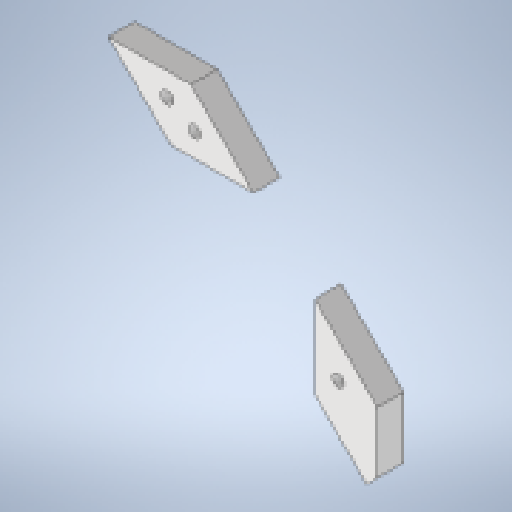
# Autodesk Inventor part: Dribbler_v1
Saved by Autodesk Inventor 2025.1 (Build 291241000, 241)
## iProperties
Created: 2026-05-04
Part Number: Dribbler_v1
Material: Generic
Document SubType Name: Modeling
Designer: User
Density: 1 g/cm^3
Appearance: Default
Author: User
## iProperties of the stored document Dribbler_v1_3DPrint.ipt
Created: 2026-05-05
Part Number: Dribbler_v1_3DPrint
Material: Generic
Document SubType Name: Modeling
Designer: User
Density: 1 g/cm^3
Appearance: Default
Author: User
Autodesk Inventor part; units mm, degrees
ref_plane "YZ Plane" through (0, 0, 0) normal (1, 0, 0) x (0, 1, 0)
ref_plane "XZ Plane" through (0, 0, 0) normal (0, 1, 0) x (-1, 0, 0)
ref_plane "XY Plane" through (0, 0, 0) normal (0, 0, 1) x (1, 0, 0)
sketch "Sketch1" plane through (0, 0, 0) normal (0, 0, 1) x (1, 0, 0)
  circle A0 centre (-1.926, 3.4009) radius 1.5 projected
  circle A1 centre (1.926, -3.4009) radius 1.5 projected
  line L0 (5.5, -12.5711) -> (5.5, 1.5711) projected
  line L1 (5.5, 1.5711) -> (-5.5, 12.5711) projected
  line L2 (-5.5, 12.5711) -> (-5.5, -1.5711) projected
  line L3 (-5.5, -1.5711) -> (5.5, -12.5711) projected
  circle A2 centre (-44.1118, 42.6369) radius 1.5 projected
  circle A3 centre (-37.31, 38.7849) radius 1.5 projected
  line L4 (-53.282, 46.2109) -> (-42.282, 35.2109) projected
  line L5 (-42.282, 35.2109) -> (-28.1398, 35.2109) projected
  line L6 (-28.1398, 35.2109) -> (-39.1398, 46.2109) projected
  line L7 (-39.1398, 46.2109) -> (-53.282, 46.2109) projected
  line L8 (-5.7, 13.0539) -> (5.7, 1.6539)
  line L9 (5.7, 1.6539) -> (5.7, -13.0539)
  line L10 (5.7, -13.0539) -> (-5.7, -1.6539)
  line L11 (-5.7, -1.6539) -> (-5.7, 13.0539)
  line L12 (-27.657, 35.0109) -> (-42.3648, 35.0109)
  line L13 (-42.3648, 35.0109) -> (-53.7648, 46.4109)
  line L14 (-53.7648, 46.4109) -> (-39.057, 46.4109)
  line L15 (-39.057, 46.4109) -> (-27.657, 35.0109)
  line L16 (-7.7, -2.4823) -> (7.7, -17.8823)
  line L17 (7.7, -17.8823) -> (7.7, 2.4823)
  line L18 (7.7, 2.4823) -> (-7.7, 17.8823)
  line L19 (-7.7, 17.8823) -> (-7.7, -2.4823)
  line L20 (-43.1932, 33.0109) -> (-22.8285, 33.0109)
  line L21 (-22.8285, 33.0109) -> (-38.2285, 48.4109)
  line L22 (-38.2285, 48.4109) -> (-58.5932, 48.4109)
  line L23 (-58.5932, 48.4109) -> (-43.1932, 33.0109)
  point P0 (0, 0)
  dimension "d0" = 0.2
  dimension "d1" = 0.2
  dimension "d2" = 2
  dimension "d3" = 2
  constraints: 32 end point, 12 other
  measures "d0" distance between parallel lines of L1 L8
  measures "d1" distance between parallel lines of L5 L12
  measures "d2" distance between parallel lines of L10 L16
  measures "d3" distance between parallel lines of L12 L20
ref_plane "Work Plane1" through (-5.5, -57.7526, -4) normal (0, 0, 1) x (1, 0, 0)
extrude "Extrusion1" add sketch "Sketch1" against normal up to surface (4 mm away) contours L19 L18 L17 L16 | L23 L22 L21 L20
sketch "Sketch2" plane through (0, 0, 0) normal (0, 0, 1) x (1, 0, 0)
  line L0 (-7.7, 17.8823) -> (-7.7, -2.4823) projected
  line L1 (7.7, 2.4823) -> (-7.7, 17.8823) projected
  line L2 (-7.7, -2.4823) -> (7.7, -17.8823) projected
  line L3 (7.7, -17.8823) -> (7.7, 2.4823) projected
  line L4 (-43.1932, 33.0109) -> (-22.8285, 33.0109) projected
  line L5 (-58.5932, 48.4109) -> (-43.1932, 33.0109) projected
  line L6 (-22.8285, 33.0109) -> (-38.2285, 48.4109) projected
  line L7 (-38.2285, 48.4109) -> (-58.5932, 48.4109) projected
  point P0 (0, 0)
extrude "Extrusion2" add sketch "Sketch2" along normal blind 2.5
sketch "Sketch3" plane through (0, 0, 2.5) normal (0, 0, 1) x (1, 0, 0)
  circle A0 centre (-44.1118, 42.6369) radius 1.5 projected
  circle A1 centre (-37.31, 38.7849) radius 1.5 projected
  circle A2 centre (-1.926, 3.4009) radius 1.5 projected
  point P0 (0, 0)
extrude "Extrusion3" cut sketch "Sketch3" against normal blind 2.5
sketch "Sketch34" plane through (0, 0, 2.5) normal (0, 0, 1) x (1, 0, 0)
  line L0 (12.8478, -6.0634) -> (8.0273, -10.8596)
  line L1 (7.7, -17.8823) -> (7.7, 2.4823) projected
  line L2 (-7.7, -2.4823) -> (7.7, -17.8823) projected
  line L3 (13.5531, -6.7723) -> (8.7326, -11.5685)
  line L4 (7.7, -12.5958) -> (5.0567, -15.2391)
  point P0 (0, 0)
  dimension "d105" = 1
  constraints: 6 end point, 2 point on line, 1 parallel, 1 perpendicular, 3 other
  measures "d105" distance between parallel lines of L0 L3
extrude "Extrusion31" cut sketch "Sketch34" against normal blind 10
sketch "Sketch36" plane through (0, 0, 2.5) normal (0, 0, 1) x (1, 0, 0)
  circle A0 centre (1.926, -3.4009) radius 1.5
  point P0 (0, 0)
  constraints: 1 centre point, 2 other
extrude "Extrusion32" cut sketch "Sketch36" against normal blind 10
sketch "Sketch37" plane through (-7.7, 17.8823, 2.5) normal (0.7071068, 0.7071068, 0) x (0, 0, -1)
  line L0 (1.1916, -14.1408) -> (1.1916, -32.4408)
  line L1 (1.6916, -14.1408) -> (1.6916, -32.4408)
  line L2 (6.5, -21.7789) -> (0, -21.7789) projected
  line L3 (6.5, 0) -> (6.5, -21.7789) projected
  line L4 (1.3722, -14.1408) -> (4.885, -14.1408)
  line L5 (1.6916, -21.7789) -> (6.5, -21.7789)
  line L6 (6.5, -21.7789) -> (6.5, -14.1408)
  line L7 (6.5, -14.1408) -> (1.6916, -14.1408)
  line L8 (1.6916, -14.1408) -> (1.6916, -21.7789)
  point P0 (2.5, -18.0894)
  point P1 (4.885, -14.1408)
  dimension "d110" = 0.5
  constraints: 14 end point, 3 parallel, 3 point on line, 2 horizontal, 1 perpendicular, 1 vertical, 4 other
  measures "d110" distance between parallel lines of L0 L1
extrude "Extrusion33" add sketch "Sketch37" along normal blind 19
sketch "Sketch38" plane through (7.7, 2.4823, -4) normal (0.7071068, -0.7071068, 0) x (0.7071068, 0.7071068, 0)
  line L0 (16.4612, 13.1005) -> (7.0738, 5.3084)
  line L1 (16.7806, 12.7158) -> (7.3931, 4.9237)
  line L2 (0, 4.8084) -> (19, 4.8084) projected
  line L3 (7.3931, 4.9237) -> (7.2543, 4.8084)
  line L4 (0, 4.8084) -> (19, 4.8084) projected
  line L5 (19, 4.8084) -> (19, 0) projected
  line L6 (16.4612, 13.1005) -> (19.5269, 9.4071)
  line L7 (19, 4.8084) -> (19, 10.0419)
  line L8 (19, 4.8084) -> (24.2335, 4.8084) construction
  arc A0 (14.4327, 6.933) -> (13.5093, 6.1666) centre (13.46, 7.1654) ccw
  circle A1 centre (13.46, 7.1654) radius 1
  point P0 (-7.2, 4)
  point P1 (14.4327, 6.933)
  point P2 (13.5093, 6.1666)
  dimension "d113" = 0.5
  dimension "d114" = 90
  constraints: 12 end point, 2 centre point, 2 point on circle, 2 point on line, 1 coincident, 1 concentric, 1 horizontal, 1 parallel, 1 perpendicular, 9 other
  measures "d113" distance between parallel lines of L0 L1
  measures "d114" angle of L8 L7
extrude "Extrusion34" add sketch "Sketch38" against normal up to surface (7.6381 mm away)
sketch "Sketch39" plane through (7.7, 2.4823, -4) normal (0.7071068, -0.7071068, 0) x (0.7071068, 0.7071068, 0)
  line L0 (7.0738, 5.3084) -> (-7.4246, 22.7752)
  line L1 (6.6891, 4.9891) -> (-7.8093, 22.4559)
  line L2 (0, 4.8084) -> (7.2543, 4.8084) projected
  line L3 (0, 4.8084) -> (0, 6.5) projected
  line L4 (-10.6619, 6.5) -> (0, 6.5) projected
  line L5 (6.6891, 4.9891) -> (6.839, 4.8084)
  line L6 (-4.6571, 4) -> (-4.6571, -2.5)
  line L7 (-4.6571, 6.5) -> (-4.6571, 4) projected
  line L8 (-4.6571, 4.8084) -> (-4.6571, 18.6583)
  point P0 (-7.2, 4)
  point P1 (-4.6571, 6.5)
  dimension "d117" = 0.5
  constraints: 10 end point, 3 point on line, 1 collinear, 1 parallel, 1 vertical, 5 other
  measures "d117" distance between parallel lines of L0 L1
extrude "Extrusion35" add sketch "Sketch39" against normal up to surface (7.6381 mm away)
sketch "Sketch40" plane through (0, 0, 2.5) normal (0, 0, 1) x (1, 0, 0)
  circle A0 centre (-1.926, 3.4009) radius 1.5 projected
  point P0 (0, 0)
  point P1 (-0.8654, 4.4616)
  constraints: 1 other
ref_plane "Work Plane4" through (-5.5, -12.5711, 0) normal (0, 0, 1) x (1, 0, 0)
extrude "Extrusion36" add sketch "Sketch40" against normal up to surface (2.5 mm away)
sketch "Sketch41" plane through (2.299, 7.8833, 2.5) normal (-0.7071068, 0.7071068, 0) x (0.7071068, 0.7071068, 0)
  line L0 (-7.4246, -16.2752) -> (1.9629, -24.0673)
  line L1 (-7.7439, -16.6599) -> (1.6435, -24.452)
  line L2 (6.839, 1.6916) -> (-4.6571, -12.1583) projected
  line L3 (-4.6571, -12.1583) -> (-4.6571, 0) projected
  line L4 (-4.6571, -12.1583) -> (-8.1286, -16.3406)
  line L5 (-8.1286, -16.3406) -> (-7.7439, -16.6599)
  arc A0 (-4.4727, -23.2091) -> (-5.396, -22.4427) centre (-4.4234, -22.2103) ccw
  circle A1 centre (-4.4234, -22.2103) radius 1
  line L6 (-5.3349, -24.2479) -> (-1.1029, -27.7607)
  line L7 (-10.4903, -19.9686) -> (-6.2583, -23.4814)
  line L8 (-5.9736, -25.0173) -> (-1.7416, -28.5301)
  line L9 (-11.129, -20.7381) -> (-6.897, -24.2509)
  line L10 (-1.1029, -27.7607) -> (1.9629, -24.0673)
  line L11 (1.6435, -24.452) -> (-1.7416, -28.5301)
  line L12 (-1.7416, -28.5301) -> (-11.5137, -20.4187)
  line L13 (0, 0) -> (-14.4, 0) projected
  line L14 (-11.5137, -20.4187) -> (-11.5137, 0)
  point P0 (-7.2, 2.5)
  point P1 (-4.4727, -23.2091)
  point P2 (-5.396, -22.4427)
  point P3 (-11.129, -20.7381)
  point P4 (-6.897, -24.2509)
  point P5 (-5.9736, -25.0173)
  point P6 (-1.1029, -27.7607)
  dimension "d122" = 0.5
  dimension "d123" = 1
  dimension "d124" = 1
  constraints: 24 end point, 4 perpendicular, 3 parallel, 2 centre point, 2 point on circle, 1 coincident, 1 concentric, 1 point on line, 14 other
  measures "d122" distance between parallel lines of L0 L1
  measures "d123" distance between parallel lines of L6 L8
  measures "d124" distance between parallel lines of L7 L9
extrude "Extrusion37" add sketch "Sketch41" against normal up to surface (7.6381 mm away)
sketch "Sketch42" plane through (0, 0, 2.5) normal (0, 0, 1) x (1, 0, 0)
  arc A0 (0.8121, -4.4055) -> (2.9306, -2.287) centre (1.926, -3.4009) ccw projected
  circle A1 centre (1.926, -3.4009) radius 3
  line L0 (0.8121, -4.4055) -> (-0.4414, -5.6591) projected
  line L1 (-0.4414, -5.6591) -> (-5.8424, -0.2581) projected
  line L2 (1.926, -3.4009) -> (4.0473, -5.5222)
  line L3 (1.926, -3.4009) -> (4.926, -3.4009) construction
  line L4 (4.0473, -5.5222) -> (-0.1953, -1.2796)
  line L5 (-0.1953, -1.2796) -> (-2.5081, -3.5924)
  point P0 (0, 0)
  point P1 (2.9867, -4.4616)
  dimension "d127" = 6
  dimension "d128" = 45
  constraints: 8 end point, 3 point on line, 2 point on circle, 1 centre point, 1 coincident, 1 equal length, 1 horizontal, 1 tangent
  measures "d127" diameter of A1
  measures "d128" angle of L2 L3
extrude "Extrusion38" cut sketch "Sketch42" along normal through all contours L0 A1 L4 L2 A0 | L2 L4 A1 | L0 L1 L5 A1
sketch "Sketch43" plane through (-5.8424, -0.2581, 22.9187) normal (-0.4516248, -0.4516248, 0.7694609) x (0.544091, 0.544091, 0.638694)
  line L0 (8.1483, -7.6381) -> (12.7, -7.6381) projected
  line L1 (0, -4.7154) -> (4.2508, -4.7154) projected
  line L2 (12.7, -7.6381) -> (0, -7.6381)
  line L3 (0, -7.6381) -> (0, -4.7154)
  line L4 (0, -4.7154) -> (12.7, -4.7154)
  line L5 (12.7, -4.7154) -> (12.7, -7.6381)
  point P0 (-11.3188, -3.9487)
  point P1 (8.1483, -7.6381)
  point P2 (4.2508, -4.7154)
  constraints: 8 end point, 2 parallel, 1 horizontal, 1 perpendicular
extrude "Extrusion39" cut sketch "Sketch43" against normal blind 10
sketch "Sketch44" plane through (2.299, 7.8833, 2.5) normal (-0.7071068, 0.7071068, 0) x (0.7071068, 0.7071068, 0)
  line L0 (-11.5137, 0) -> (-11.5137, -20.4187) projected
  line L1 (0, 0) -> (-14.4, 0) projected
  line L2 (-11.5137, -20.4187) -> (-1.7416, -28.5301) projected
  line L3 (-14.4, 6.5) -> (-14.4, 0) projected
  line L4 (-14.4, 0) -> (-14.4, -18.023)
  line L5 (-14.4, -18.023) -> (-11.5137, -20.4187)
  point P0 (-7.2, 2.5)
  constraints: 4 end point, 1 vertical
extrude "Extrusion40" add sketch "Sketch44" against normal up to surface (4.7154 mm away)
sketch "Sketch45" plane through (0, 0, 2.5) normal (0, 0, 1) x (1, 0, 0)
  line L0 (-7.8833, -2.299) -> (1.0675, 6.6518) projected
  line L1 (-7.7, 17.8823) -> (-7.7, -2.1157) projected
  line L2 (-1.5165, 4.0677) -> (-3.4257, 5.9769)
  line L3 (-1.5165, 4.0677) -> (-3.6379, 1.9464)
  line L4 (-3.6379, 1.9464) -> (-9.8213, 8.1299)
  line L5 (-9.8213, 8.1299) -> (-7.7, 10.2512)
  line L6 (-7.7, 10.2512) -> (-1.5165, 4.0677)
  point P0 (0, 0)
  point P1 (-7.7, 6.0086)
  dimension "d135" = 3
  constraints: 10 end point, 2 parallel, 1 perpendicular, 1 point on line, 3 other
  measures "d135" distance of L2.start L3.end
extrude "Extrusion41" add sketch "Sketch45" along normal up to surface contours L4 L1 L6 L2 L0 surface through (4.4069, -0.8107, 14.6583) normal (0.544091, 0.544091, 0.638694)
sketch "Sketch46" plane through (-7.7, -2.4823, -4) normal (0, 0, -1) x (-1, 0, 0)
  line L0 (0, 0) -> (0, 20.3647) projected
  line L1 (-2, 15.5362) -> (-2, 0.8284) projected
  line L2 (-12.7567, -12.7567) -> (0, 0) projected
  line L3 (0, 20.3647) -> (-9.999, 10.3657) projected
  line L4 (-2.0031, 18.3616) -> (-2, -2)
  line L5 (35.4932, 35.4932) -> (50.8932, 50.8932) projected
  line L6 (15.1285, 35.4932) -> (35.4932, 35.4932) projected
  line L7 (34.6648, 37.4932) -> (19.957, 37.4932) projected
  line L8 (30.5285, 50.8932) -> (15.1285, 35.4932) projected
  line L9 (37.4692, 37.4692) -> (17.1285, 37.4932)
  point P0 (-7.7, 2.4823)
  constraints: 6 point on line, 4 end point
extrude "Extrusion42" add sketch "Sketch46" along normal blind 5
sketch "Sketch47" plane through (0, 0, 2.5) normal (0, 0, 1) x (1, 0, 0)
  line L0 (5.5, -57.7526) -> (5.5, -12.5711)
  line L1 (-7.7, 6.0086) -> (-7.7, -2.1157) projected
  line L2 (-4.549, -5.6333) -> (5.0567, -15.2391) projected
  line L3 (5.0567, -15.2391) -> (5.0567, -34.2391)
  line L4 (5.0567, -34.2391) -> (-7.7, -34.2391)
  line L5 (-7.7, -34.2391) -> (-7.7, -2.1157)
  line L6 (5.0567, -15.2391) -> (7.7, -12.5958) projected
  line L7 (-7.8833, -2.299) -> (-4.549, -5.6333) projected
  point P0 (0, 0)
  point P1 (-7.7, -2.4823)
  dimension "d140" = 19
  dimension "d141" = 90
  constraints: 8 end point, 1 collinear, 1 parallel, 1 vertical, 2 other
  measures "d140" distance of L2.end L3.end
  measures "d141" angle of L3 L4
extrude "Extrusion43" add sketch "Sketch47" against normal up to surface (6.5 mm away)
sketch "Sketch48" plane through (0, 0, 2.5) normal (0, 0, 1) x (1, 0, 0)
  line L0 (-53.282, 46.2109) -> (-98.4635, 46.2109)
  line L1 (-38.2285, 48.4109) -> (-58.5932, 48.4109) projected
  line L2 (-58.5932, 48.4109) -> (-43.1932, 33.0109) projected
  line L3 (-56.3932, 46.2109) -> (-54.1932, 48.4109)
  line L4 (-56.3932, 46.2109) -> (-53.282, 46.2109) construction
  line L5 (-56.3932, 46.2109) -> (-55.6861, 45.5038)
  line L6 (-55.6861, 45.5038) -> (-52.779, 48.4109)
  point P0 (0, 0)
  dimension "d144" = 45
  dimension "d145" = 1
  constraints: 10 end point, 5 point on line, 2 horizontal, 1 equal length, 1 perpendicular, 2 other
  measures "d144" angle of L4 L3
  measures "d145" distance of L3.start L5.end
extrude "Extrusion44" cut sketch "Sketch48" against normal blind 10
sketch "Sketch50" plane through (0, 0, 2.5) normal (0, 0, 1) x (1, 0, 0)
  line L0 (-43.1932, 33.0109) -> (-22.8285, 33.0109) projected
  line L1 (-55.6861, 45.5038) -> (-43.1932, 33.0109) projected
  line L2 (-53.282, 46.2109) -> (-98.4635, 46.2109)
  line L3 (-7.7, -2.4823) -> (-7.7, -34.2391) projected
  line L4 (-55.6861, 45.5038) -> (-88.933, 45.5038)
  line L5 (-7.7, -34.2391) -> (-87.4429, 45.5038)
  line L6 (-7.7, -34.2391) -> (105.0734, -34.2391) construction
  line L7 (-22.8285, 33.0109) -> (-74.95, 33.0109)
  point P0 (0, 0)
  dimension "d148" = 135
  constraints: 10 end point, 3 horizontal, 2 point on line, 1 equal length, 1 parallel, 2 other
  measures "d148" angle of L6 L5
extrude "Extrusion45" add sketch "Sketch50" against normal up to surface (6.5 mm away)
sketch "Sketch51" plane through (0, 0, 2.5) normal (0, 0, 1) x (1, 0, 0)
  line L0 (-7.7, -34.2391) -> (5.0567, -34.2391) projected
  line L1 (-87.4429, 45.5038) -> (-74.95, 33.0109) projected
  line L2 (-7.7, -34.2391) -> (5.0567, -46.9958)
  line L3 (-7.7, -34.2391) -> (10.3408, -34.2391) construction
  line L4 (5.0567, -46.9958) -> (5.0567, -34.2391)
  point P0 (0, 0)
  dimension "d151" = 45
  constraints: 6 end point, 1 equal length, 1 horizontal
  measures "d151" angle of L2 L3
ref_plane "Work Plane5" through (-5.5, -57.7526, -4) normal (0, 0, 1) x (1, 0, 0)
extrude "Extrusion46" add sketch "Sketch51" against normal up to surface (6.5 mm away)
sketch "Sketch52" plane through (-38.2285, 48.4109, -4) normal (0, 0, -1) x (-1, 0, 0)
  line L0 (4.9647, -15.4) -> (36.7214, -15.4) projected
  line L1 (6.9407, -13.424) -> (-13.4, -13.4) projected
  line L2 (36.7214, -15.4) -> (49.2143, -2.9071) projected
  line L3 (4.9647, -15.4) -> (6.9407, -13.424) projected
  line L4 (6.9407, -13.424) -> (38.6974, -13.424)
  line L5 (-30.5285, -82.65) -> (-30.5285, -50.8932) projected
  line L6 (-32.5285, -52.8932) -> (-30.5285, -50.8932) projected
  line L7 (-43.2853, -95.4067) -> (-30.5285, -82.65) projected
  line L8 (-32.5285, -52.8932) -> (-32.5285, -84.65)
  point P0 (-38.2285, -48.4109)
  constraints: 4 end point, 2 point on line, 1 parallel, 1 vertical
extrude "Extrusion47" add sketch "Sketch52" along normal up to surface (5 mm away)
sketch "Sketch53" plane through (-7.7, -34.2391, 2.5) normal (-0.7071068, -0.7071068, 0) x (-0.7071068, 0.7071068, 0)
  line L0 (0, 0) -> (-18.0408, 0) projected
  line L1 (112.7734, 0) -> (95.1058, 0) projected
  line L2 (95.1058, 0) -> (95.1058, -15)
  line L3 (0, 0) -> (0, 11.5) projected
  line L4 (0, 0) -> (0, -15)
  line L5 (-6, 0) -> (-6, -15)
  line L6 (101.1058, -15) -> (101.1058, 0)
  line L7 (101.1058, -15) -> (95.1058, -15)
  line L8 (0, -15) -> (-6, -15)
  point P0 (18.766, 2.5)
  point P1 (-6, 0)
  dimension "d156" = 15
  dimension "d157" = 15
  dimension "d158" = 6
  dimension "d159" = 6
  constraints: 12 end point, 2 equal length, 2 vertical, 1 horizontal, 1 perpendicular, 1 point on line
  measures "d156" distance of L1.end L2.end
  measures "d157" distance of L0.start L4.end
  measures "d158" distance between parallel lines of L4 L5
  measures "d159" distance between parallel lines of L2 L6
extrude "Extrusion48" add sketch "Sketch53" against normal up to surface surface through (-87.4429, 45.5038, 2.5) normal (0, 1, 0)
sketch "Sketch54" plane through (5.0567, -29.9676, 2.5) normal (0, 0, -1) x (-1, 0, 0)
  line L0 (0, 0) -> (0, 8.4853) projected
  line L1 (0, 8.4853) -> (-66.9861, 75.4714) projected
  line L2 (-66.9861, 75.4714) -> (-75.4714, 75.4714) projected
  line L3 (0, 0) -> (-75.4714, 75.4714) projected
  point P0 (5.0567, 29.9676)
extrude "Extrusion49" cut sketch "Sketch54" against normal through all
sketch "Sketch55" plane through (-79.1926, 37.2535, 2.5) normal (-0.7071068, 0.7071068, 0) x (-0.7071068, -0.7071068, 0)
  line L0 (0, 15) -> (-11.6676, 15) projected
  line L1 (0, 15) -> (0, 0) projected
  line L2 (-11.6676, 15) -> (-11.6676, 0) projected
  line L3 (0, 15) -> (-11.6676, 15)
  line L4 (-11.6676, 15) -> (-11.6676, 3.332)
  line L5 (-11.6676, 3.332) -> (0, 3.332)
  line L6 (0, 3.332) -> (0, 15)
  line L7 (-11.6676, 3.332) -> (0, 15)
  circle A0 centre (-5.8338, 9.166) radius 1.6
  point P0 (-29.6554, -2.5)
  dimension "d164" = 11.668
  dimension "d165" = 3.2
  constraints: 10 end point, 2 parallel, 1 centre point, 1 horizontal, 1 midpoint, 1 perpendicular, 1 point on line
  measures "d164" distance of L4.end L3.end
  measures "d165" diameter of A0
extrude "Extrusion50" cut sketch "Sketch55" against normal through all contours A0 L7 | L7 A0
body "Solid1"
